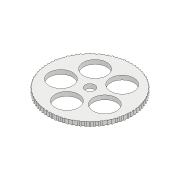
# Autodesk Inventor part: Polea Dentada Grande
Saved by Autodesk Inventor 2020 (Build 240168000, 168)
## iProperties
Part Number: Polea Dentada Grande
Material: Genérico
Document SubType Name: Modeling
Designer: FABLAB
Density: 1 g/cm^3
Appearance: Blanco
Author: FABLAB
Autodesk Inventor part; units mm, degrees
ref_plane "YZ Plane" through (0, 0, 0) normal (1, 0, 0) x (0, 1, 0)
ref_plane "XZ Plane" through (0, 0, 0) normal (0, 1, 0) x (-1, 0, 0)
ref_plane "XY Plane" through (0, 0, 0) normal (0, 0, 1) x (1, 0, 0)
sketch "Boceto1" plane through (0, 0, 0) normal (0, 0, 1) x (1, 0, 0)
  arc A0 (53.777, -26.6088) -> (-59.9943, 0.8261) centre (0, 0) ccw
  circle A1 centre (60, 0) radius 1
  arc A2 (-62.4245, -175.6651) -> (-24.5007, -184.8101) centre (-42.4264, -175.9405) ccw construction
  line L0 (-24.5007, -184.8101) -> (53.777, -26.6088) construction
  line L1 (-62.4245, -175.6651) -> (-59.9943, 0.8261) construction
  circle A3 centre (59.815, 4.7075) radius 1
  circle A4 centre (59.2613, 9.3861) radius 1
  circle A5 centre (58.3422, 14.0067) radius 1
  circle A6 centre (57.0634, 18.541) radius 1
  circle A7 centre (55.4328, 22.961) radius 1
  circle A8 centre (53.4604, 27.2394) radius 1
  circle A9 centre (51.1584, 31.3499) radius 1
  circle A10 centre (48.541, 35.2671) radius 1
  circle A11 centre (45.6244, 38.9669) radius 1
  circle A12 centre (42.4264, 42.4264) radius 1
  circle A13 centre (38.9669, 45.6244) radius 1
  circle A14 centre (35.2671, 48.541) radius 1
  circle A15 centre (31.3499, 51.1584) radius 1
  circle A16 centre (27.2394, 53.4604) radius 1
  circle A17 centre (22.961, 55.4328) radius 1
  circle A18 centre (18.541, 57.0634) radius 1
  circle A19 centre (14.0067, 58.3422) radius 1
  circle A20 centre (9.3861, 59.2613) radius 1
  circle A21 centre (4.7075, 59.815) radius 1
  circle A22 centre (0, 60) radius 1
  circle A23 centre (-4.7075, 59.815) radius 1
  circle A24 centre (-9.3861, 59.2613) radius 1
  circle A25 centre (-14.0067, 58.3422) radius 1
  circle A26 centre (-18.541, 57.0634) radius 1
  circle A27 centre (-22.961, 55.4328) radius 1
  circle A28 centre (-27.2394, 53.4604) radius 1
  circle A29 centre (-31.3499, 51.1584) radius 1
  circle A30 centre (-35.2671, 48.541) radius 1
  circle A31 centre (-38.9669, 45.6244) radius 1
  circle A32 centre (-42.4264, 42.4264) radius 1
  circle A33 centre (-45.6244, 38.9669) radius 1
  circle A34 centre (-48.541, 35.2671) radius 1
  circle A35 centre (-51.1584, 31.3499) radius 1
  circle A36 centre (-53.4604, 27.2394) radius 1
  circle A37 centre (-55.4328, 22.961) radius 1
  circle A38 centre (-57.0634, 18.541) radius 1
  circle A39 centre (-58.3422, 14.0067) radius 1
  circle A40 centre (-59.2613, 9.3861) radius 1
  circle A41 centre (-59.815, 4.7075) radius 1
  circle A42 centre (-60, 0) radius 1
  circle A43 centre (-59.815, -4.7075) radius 1
  circle A44 centre (-59.2613, -9.3861) radius 1
  circle A45 centre (-58.3422, -14.0067) radius 1
  circle A46 centre (-57.0634, -18.541) radius 1
  circle A47 centre (-55.4328, -22.961) radius 1
  circle A48 centre (-53.4604, -27.2394) radius 1
  circle A49 centre (-51.1584, -31.3499) radius 1
  circle A50 centre (-48.541, -35.2671) radius 1
  circle A51 centre (-45.6244, -38.9669) radius 1
  circle A52 centre (-42.4264, -42.4264) radius 1
  circle A53 centre (-38.9669, -45.6244) radius 1
  circle A54 centre (-35.2671, -48.541) radius 1
  circle A55 centre (-31.3499, -51.1584) radius 1
  circle A56 centre (-27.2394, -53.4604) radius 1
  circle A57 centre (-22.961, -55.4328) radius 1
  circle A58 centre (-18.541, -57.0634) radius 1
  circle A59 centre (-14.0067, -58.3422) radius 1
  circle A60 centre (-9.3861, -59.2613) radius 1
  circle A61 centre (-4.7075, -59.815) radius 1
  circle A62 centre (0, -60) radius 1
  circle A63 centre (4.7075, -59.815) radius 1
  circle A64 centre (9.3861, -59.2613) radius 1
  arc A65 (-59.9943, 0.8261) -> (53.777, -26.6088) centre (0, 0) ccw construction
  circle A66 centre (0, 0) radius 60
  circle A67 centre (14.0067, -58.3422) radius 1
  circle A68 centre (18.541, -57.0634) radius 1
  circle A69 centre (22.961, -55.4328) radius 1
  circle A70 centre (27.2394, -53.4604) radius 1
  circle A71 centre (31.3499, -51.1584) radius 1
  circle A72 centre (35.2671, -48.541) radius 1
  circle A73 centre (38.9669, -45.6244) radius 1
  circle A74 centre (42.4264, -42.4264) radius 1
  circle A75 centre (45.6244, -38.9669) radius 1
  circle A76 centre (48.541, -35.2671) radius 1
  circle A77 centre (51.1584, -31.3499) radius 1
  circle A78 centre (53.4604, -27.2394) radius 1
  circle A79 centre (55.4328, -22.961) radius 1
  circle A80 centre (57.0634, -18.541) radius 1
  circle A81 centre (58.3422, -14.0067) radius 1
  circle A82 centre (59.2613, -9.3861) radius 1
  circle A83 centre (59.815, -4.7075) radius 1
  circle A84 centre (0, 0) radius 7
  circle A85 centre (0, -33.5) radius 16.8954
  line L2 (0, -7) -> (0, -60) construction
  circle A86 centre (31.8604, -10.3521) radius 16.8954
  circle A87 centre (19.6908, 27.1021) radius 16.8954
  circle A88 centre (-19.6908, 27.1021) radius 16.8954
  circle A89 centre (-31.8604, -10.3521) radius 16.8954
  point P0 (53.9069, -26.3447)
  point P1 (55.0424, -23.8817)
  point P2 (55.8077, -22.034)
  point P3 (56.7465, -19.4895)
  point P4 (57.3645, -17.5874)
  point P5 (58.1007, -14.9771)
  point P6 (58.5675, -13.0324)
  point P7 (59.0966, -10.3724)
  point P8 (59.4095, -8.3971)
  point P9 (59.7283, -5.7038)
  point P10 (59.8852, -3.71)
  point P11 (59.9917, -1)
  point P12 (59.9917, 1)
  point P13 (59.8852, 3.71)
  point P14 (59.7283, 5.7038)
  point P15 (59.4095, 8.3971)
  point P16 (59.0966, 10.3724)
  point P17 (58.5675, 13.0324)
  point P18 (58.1007, 14.9771)
  point P19 (57.3645, 17.5874)
  point P20 (56.7465, 19.4895)
  point P21 (55.8077, 22.034)
  point P22 (55.0424, 23.8817)
  point P23 (53.9069, 26.3447)
  point P24 (52.999, 28.1266)
  point P25 (51.6738, 30.4929)
  point P26 (50.6288, 32.1982)
  point P27 (49.122, 34.4532)
  point P28 (47.9465, 36.0712)
  point P29 (46.2674, 38.2011)
  point P30 (44.9686, 39.7219)
  point P31 (43.1276, 41.7134)
  point P32 (41.7134, 43.1276)
  point P33 (39.7219, 44.9686)
  point P34 (38.2011, 46.2674)
  point P35 (36.0712, 47.9465)
  point P36 (34.4532, 49.122)
  point P37 (32.1982, 50.6288)
  point P38 (30.4929, 51.6738)
  point P39 (28.1266, 52.999)
  point P40 (26.3447, 53.9069)
  point P41 (23.8817, 55.0424)
  point P42 (22.034, 55.8077)
  point P43 (19.4895, 56.7465)
  point P44 (17.5874, 57.3645)
  point P45 (14.9771, 58.1007)
  point P46 (13.0324, 58.5675)
  point P47 (10.3724, 59.0966)
  point P48 (8.3971, 59.4095)
  point P49 (5.7038, 59.7283)
  point P50 (3.71, 59.8852)
  point P51 (1, 59.9917)
  point P52 (-1, 59.9917)
  point P53 (-3.71, 59.8852)
  point P54 (-5.7038, 59.7283)
  point P55 (-8.3971, 59.4095)
  point P56 (-10.3724, 59.0966)
  point P57 (-13.0324, 58.5675)
  point P58 (-14.9771, 58.1007)
  point P59 (-17.5874, 57.3645)
  point P60 (-19.4895, 56.7465)
  point P61 (-22.034, 55.8077)
  point P62 (-23.8817, 55.0424)
  point P63 (-26.3447, 53.9069)
  point P64 (-28.1266, 52.999)
  point P65 (-30.4929, 51.6738)
  point P66 (-32.1982, 50.6288)
  point P67 (-34.4532, 49.122)
  point P68 (-36.0712, 47.9465)
  point P69 (-38.2011, 46.2674)
  point P70 (-39.7219, 44.9686)
  point P71 (-41.7134, 43.1276)
  point P72 (-43.1276, 41.7134)
  point P73 (-44.9686, 39.7219)
  point P74 (-46.2674, 38.2011)
  point P75 (-47.9465, 36.0712)
  point P76 (-49.122, 34.4532)
  point P77 (-50.6288, 32.1982)
  point P78 (-51.6738, 30.4929)
  point P79 (-52.999, 28.1266)
  point P80 (-53.9069, 26.3447)
  point P81 (-55.0424, 23.8817)
  point P82 (-55.8077, 22.034)
  point P83 (-56.7465, 19.4895)
  point P84 (-57.3645, 17.5874)
  point P85 (-58.1007, 14.9771)
  point P86 (-58.5675, 13.0324)
  point P87 (-59.0966, 10.3724)
  point P88 (-59.4095, 8.3971)
  point P89 (-59.7283, 5.7038)
  point P90 (-59.8852, 3.71)
  point P91 (-59.9917, 1)
  point P92 (-59.9917, -1)
  point P93 (-59.8852, -3.71)
  point P94 (-59.7283, -5.7038)
  point P95 (-59.4095, -8.3971)
  point P96 (-59.0966, -10.3724)
  point P97 (-58.5675, -13.0324)
  point P98 (-58.1007, -14.9771)
  point P99 (-57.3645, -17.5874)
  point P100 (-56.7465, -19.4895)
  point P101 (-55.8077, -22.034)
  point P102 (-55.0424, -23.8817)
  point P103 (-53.9069, -26.3447)
  point P104 (-52.999, -28.1266)
  point P105 (-51.6738, -30.4929)
  point P106 (-50.6288, -32.1982)
  point P107 (-49.122, -34.4532)
  point P108 (-47.9465, -36.0712)
  point P109 (-46.2674, -38.2011)
  point P110 (-44.9686, -39.7219)
  point P111 (-43.1276, -41.7134)
  point P112 (-41.7134, -43.1276)
  point P113 (-39.7219, -44.9686)
  point P114 (-38.2011, -46.2674)
  point P115 (-36.0712, -47.9465)
  point P116 (-34.4532, -49.122)
  point P117 (-32.1982, -50.6288)
  point P118 (-30.4929, -51.6738)
  point P119 (-28.1266, -52.999)
  point P120 (-26.3447, -53.9069)
  point P121 (-23.8817, -55.0424)
  point P122 (-22.034, -55.8077)
  point P123 (-19.4895, -56.7465)
  point P124 (-17.5874, -57.3645)
  point P125 (-14.9771, -58.1007)
  point P126 (-13.0324, -58.5675)
  point P127 (-10.3724, -59.0966)
  point P128 (-8.3971, -59.4095)
  point P129 (-5.7038, -59.7283)
  point P130 (-3.71, -59.8852)
  point P131 (-1, -59.9917)
  point P132 (1, -59.9917)
  point P133 (3.71, -59.8852)
  point P134 (5.7038, -59.7283)
  point P135 (8.3971, -59.4095)
  point P136 (10.3724, -59.0966)
  point P137 (13.0324, -58.5675)
  point P138 (14.9771, -58.1007)
  point P139 (17.5874, -57.3645)
  point P140 (19.4895, -56.7465)
  point P141 (22.034, -55.8077)
  point P142 (23.8817, -55.0424)
  point P143 (26.3447, -53.9069)
  point P144 (28.1266, -52.999)
  point P145 (30.4929, -51.6738)
  point P146 (32.1982, -50.6288)
  point P147 (34.4532, -49.122)
  point P148 (36.0712, -47.9465)
  point P149 (38.2011, -46.2674)
  point P150 (39.7219, -44.9686)
  point P151 (41.7134, -43.1276)
  point P152 (43.1276, -41.7134)
  point P153 (44.9686, -39.7219)
  point P154 (46.2674, -38.2011)
  point P155 (47.9465, -36.0712)
  point P156 (49.122, -34.4532)
  point P157 (50.6288, -32.1982)
  point P158 (51.6738, -30.4929)
  point P159 (52.999, -28.1266)
  point P160 (0, -33.5)
  dimension "d0" = 120
  dimension "d21" = 215.2381
  dimension "d31" = 14
  dimension "d9" = 2
  dimension "d22" = 176.5079
  dimension "d23" = 20
  dimension "d26" = 360
  dimension "d28" = 4.7112
  dimension "d34" = 360
  constraints: 87 centre point, 6 end point, 4 coincident, 4 point on circle, 4 tangent, 1 horizontal alignment, 1 midpoint, 1 point on line, 1 vertical, 1 vertical alignment, 184 other
  measures "d9" diameter of A1
  measures "d22" distance of L0.start L0.end
  measures "d23" radius of A2
  measures "d28" distance of A9.centre A10.centre
extrude "Extrusión1" add sketch "Boceto1" along normal blind 6
sketch "Boceto2" plane through (0, 0, 6) normal (0, 0, 1) x (1, 0, 0)
  circle A0 centre (0, 0) radius 41.5
  arc A1 (20.168, 17.783) -> (20.168, -17.783) centre (101.6471, 0) ccw
  arc A2 (20.168, 17.783) -> (5.3165, 26.3575) centre (11.375, 19.7021) ccw projected
  arc A3 (-25.4845, 8.5745) -> (5.3165, 26.3575) centre (-50.8235, 88.0289) ccw
  arc A4 (-25.4845, 8.5745) -> (-25.4845, -8.5745) centre (-22.75, 0) ccw
  arc A5 (5.3165, -26.3575) -> (-25.4845, -8.5745) centre (-50.8235, -88.0289) ccw projected
  arc A6 (5.3165, -26.3575) -> (20.168, -17.783) centre (11.375, -19.7021) ccw projected
  circle A7 centre (-13.375, -23.1662) radius 1.5 projected
  circle A8 centre (-13.375, 23.1662) radius 1.5 projected
  circle A9 centre (26.75, 0) radius 1.5 projected
  dimension "d30" = 83
  constraints: 6 point on circle, 4 centre point, 1 coincident, 11 other
  measures "d30" diameter of A0
sketch "Boceto3" plane through (0, 0, 0) normal (0, 0, -1) x (-1, 0, 0)
  circle A0 centre (0, 0) radius 41.5 projected
  circle A1 centre (0, 0) radius 36
  dimension "d6" = 5.5
  constraints: 1 centre point
  measures "d6" radial gap between concentric circles of A0 A1
